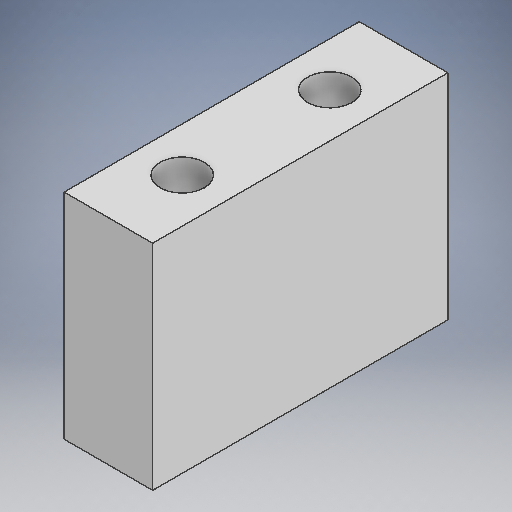
# Autodesk Inventor part: shoe_lace
Saved by Autodesk Inventor 2026.1 (Build 301233000, 233)
## iProperties
Created: 2025-12-16
Part Number: shoe_lace
Material: Generic
Document SubType Name: Modeling
Designer: emanuel
Density: 1 g/cm^3
Appearance: Default
Author: emanuel
Autodesk Inventor part; units mm, degrees
ref_plane "YZ Plane" through (0, 0, 0) normal (1, 0, 0) x (0, 1, 0)
ref_plane "XZ Plane" through (0, 0, 0) normal (0, 1, 0) x (-1, 0, 0)
ref_plane "XY Plane" through (0, 0, 0) normal (0, 0, 1) x (1, 0, 0)
sketch "Sketch1" plane through (0, 0, 0) normal (1, 0, 0) x (0, 1, 0)
  line L0 (0, 0) -> (14.5, 0)
  line L1 (14.5, 0) -> (14.5, -20)
  line L2 (14.5, -20) -> (0, -20)
  line L3 (0, -20) -> (0, 0)
  dimension "d0" = 14.5
  dimension "d1" = 20
  constraints: 8 end point, 2 parallel, 1 horizontal, 1 perpendicular
  measures "d0" distance of L1.end L2.end
  measures "d1" distance of L0.end L1.end
extrude "Extrusion1" add sketch "Sketch1" along normal blind 6
sketch "Sketch2" plane through (0, 14.5, 0) normal (0, 1, 0) x (1, 0, 0)
  line L0 (0, 0) -> (3, 0)
  line L1 (3, 0) -> (3, 5)
  line L2 (3, 5) -> (0, 5)
  line L3 (0, 5) -> (0, 0)
  line L4 (0, 20) -> (6, 20) projected
  line L5 (6, 20) -> (3, 20)
  line L6 (3, 20) -> (3, 15)
  line L7 (3, 15) -> (6, 15)
  line L8 (6, 15) -> (6, 20)
  circle A0 centre (3, 5) radius 1.5
  circle A1 centre (3, 15) radius 1.5
  dimension "d4" = 3
  dimension "d5" = 5
  dimension "d6" = 3
  dimension "d7" = 5
  dimension "d8" = 3
  dimension "d9" = 3
  constraints: 16 end point, 4 parallel, 2 centre point, 2 coincident, 2 horizontal, 2 perpendicular
  measures "d4" distance of L2.end L1.end
  measures "d5" distance of L1.end L0.end
  measures "d6" distance of L7.end L6.end
  measures "d7" distance of L6.end L5.end
  measures "d8" diameter of A0
  measures "d9" diameter of A1
extrude "Extrusion2" cut sketch "Sketch2" against normal blind 164 contours A0 L2 L1 | L1 L2 A0 | A1 L7 L6 | L6 L7 A1
body "Solid1"
